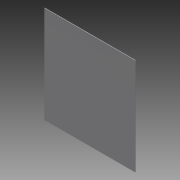
# Autodesk Inventor part: Chassis_Alu
Saved by Autodesk Inventor 2013 (Build 170138000, 138)
## iProperties
Created: 2015-07-02
Part Number: Chassis_Alu
Material: Steel
Document SubType Name: Modeling
Designer: Kyle
Density: 7.85 g/cm^3
Mass: 58.1417 g
Surface Area: 257.297 cm^2
Volume: 7.40658 cm^3
Author: Kyle
Autodesk Inventor part; units mm, degrees
ref_plane "YZ Plane" through (0, 0, 0) normal (1, 0, 0) x (0, 1, 0)
ref_plane "XZ Plane" through (0, 0, 0) normal (0, 1, 0) x (-1, 0, 0)
ref_plane "XY Plane" through (0, 0, 0) normal (0, 0, 1) x (1, 0, 0)
sketch "Sketch1" plane through (0, 0, 0) normal (0, 0, 1) x (1, 0, 0)
  line L0 (0, 0) -> (0, 116.586)
  line L1 (0, 116.586) -> (109.22, 116.586)
  line L2 (109.22, 116.586) -> (109.22, 0)
  line L3 (109.22, 0) -> (0, 0)
  dimension "d0" = 109.22
  dimension "d1" = 116.586
  constraints: 8 end point, 2 parallel, 1 perpendicular, 1 vertical
  measures "d0" distance of L2.end L0.start
  measures "d1" distance of L0.start L0.end
extrude "Extrusion1" add sketch "Sketch1" along normal blind 0.5817
body "Solid1"
